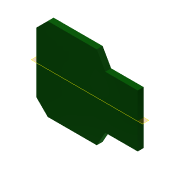
# Autodesk Inventor part: 32ch_ACF2TDT_board_3p0
Saved by Autodesk Inventor 2014 (Build 180170000, 170)
## iProperties
Created: 2016-08-28
Part Number: 32ch_ACF2TDT_board_3p0
Material: Generic
Document SubType Name: Modeling
Designer: Camilo
Density: 1 g/cm^3
Appearance: LED - Green Off
Author: Camilo
Autodesk Inventor part; units mm, degrees
ref_plane "YZ Plane" through (0, 0, 0) normal (1, 0, 0) x (0, 1, 0)
ref_plane "XZ Plane" through (0, 0, 0) normal (0, 1, 0) x (-1, 0, 0)
ref_plane "XY Plane" through (0, 0, 0) normal (0, 0, 1) x (1, 0, 0)
sketch "Sketch1" plane through (0, 0, 0) normal (0, 1, 0) x (-1, 0, 0)
  line L0 (4.3002, 1.999) -> (5.4254, 0)
  line L1 (5.4254, 0) -> (11.9253, 0)
  line L2 (11.9253, 0) -> (13.4239, 1.5011)
  line L3 (13.4239, 1.5011) -> (13.4239, 9.4996)
  line L4 (13.4239, 9.4996) -> (11.9253, 11.0007)
  line L5 (11.9253, 11.0007) -> (5.4254, 11.0007)
  line L6 (5.4254, 11.0007) -> (4.3002, 8.9992)
  line L7 (4.3002, 8.9992) -> (0, 8.9992)
  line L8 (0, 8.9992) -> (0, 1.999)
  line L9 (0, 1.999) -> (4.3002, 1.999)
  line L10 (0, 8.9992) -> (4.3002, 8.9992)
  line L11 (4.3002, 8.9992) -> (5.4254, 11.0007)
  line L12 (5.4254, 11.0007) -> (11.9253, 11.0007)
  line L13 (11.9253, 11.0007) -> (13.4239, 9.4996)
  line L14 (13.4239, 9.4996) -> (13.4239, 1.5011)
  line L15 (13.4239, 1.5011) -> (11.9253, 0)
  line L16 (11.9253, 0) -> (5.4254, 0)
  line L17 (5.4254, 0) -> (4.3002, 1.999)
  line L18 (4.3002, 1.999) -> (0, 1.999)
  line L19 (0, 1.999) -> (0, 8.9992)
  point P0 (0, 0)
  constraints: 40 end point
extrude "Extrusion1" add sketch "Sketch1" along normal blind 0.78
ref_plane "Work Plane1" through (-11.9253, 0, 5.5004) normal (0, 0, 1) x (1, 0, 0)
body "Solid1"
